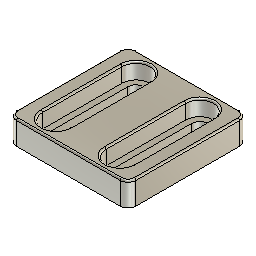
Y_stop v1_optional (Autodesk Fusion 360 design; units mm, degrees)
Autodesk Fusion 360 part; units mm, degrees
sketch "Sketch1" plane through (0, 0, 0) normal (0, 0, 1) x (1, 0, 0)
  line L0 (0, 0) -> (30, 0)
  line L1 (30, 0) -> (30, 30)
  line L2 (30, 30) -> (0, 30)
  line L3 (0, 30) -> (0, 0)
  line L4 (7, 30) -> (7, 0) construction
  line L5 (23, 30) -> (23, 0) construction
  line L6 (15, 30) -> (15, 0) construction
  line L7 (3.5, 24.986) -> (3.5, 4.986)
  line L8 (10.5, 24.986) -> (10.5, 4.986)
  arc A0 (10.5, 24.986) -> (3.5, 24.986) centre (7, 24.986) ccw
  arc A1 (3.5, 4.986) -> (10.5, 4.986) centre (7, 4.986) ccw
  line L9 (5, 24.9854) -> (5, 4.9865)
  line L10 (9, 24.986) -> (9, 4.986)
  arc A2 (9, 24.986) -> (5, 24.9854) centre (7, 24.986) ccw
  arc A3 (5, 4.9865) -> (9, 4.986) centre (7, 4.986) ccw
  line L11 (26.5, 24.986) -> (26.5, 4.986)
  line L12 (25, 24.9854) -> (25, 4.9865)
  arc A4 (25, 24.9854) -> (21, 24.986) centre (23, 24.986) ccw
  arc A5 (21, 4.986) -> (25, 4.9865) centre (23, 4.986) ccw
  arc A6 (26.5, 24.986) -> (19.5, 24.986) centre (23, 24.986) ccw
  line L13 (19.5, 24.986) -> (19.5, 4.986)
  line L14 (21, 24.986) -> (21, 4.986)
  arc A7 (19.5, 4.986) -> (26.5, 4.986) centre (23, 4.986) ccw
  point P0 (7, 21.986)
  point P1 (23, 21.9825)
  point P2 (23.0012, 7.9825)
  point P3 (7.0013, 7.986)
  point P4 (23, 21.986)
  point P5 (22.9987, 7.986)
  dimension "d1" = 30
  dimension "d2" = 30
  dimension "d3" = 16
  dimension "d4" = 14
  dimension "d5" = 7
  dimension "d6" = 3
  dimension "d7" = 14
  dimension "d8" = 16
  dimension "d9" = 7
  dimension "d10" = 3
  dimension "d11" = 7
  dimension "d12" = 4
  dimension "d13" = 4
  dimension "d14" = 4
  constraint horizontal L0
  constraint vertical L1
  constraint horizontal L2
  constraint vertical L3
  constraint coincident L0.start L3.end
  constraint parallel L1 L4
  constraint perpendicular L2 L5
  constraint coincident L2 L4.start
  constraint coincident L2 L5.start
  constraint coincident L0 L5.end
  constraint coincident L0 L4.end
  constraint coincident L4 A0.centre
  constraint coincident L4 A1.centre
  constraint midpoint L2 L6.start
  constraint midpoint L0 L6.end
  constraint perpendicular L2 L7
  constraint parallel L4 L8
  constraint symmetric L4 L7 L8
  constraint concentric A0 A2
  constraint concentric A1 A3
  constraint parallel L7 L9
  constraint parallel L4 L10
  constraint symmetric P0 L6 P4
  constraint symmetric P3 L6 P5
  constraint symmetric L6 L7.start L11.start
  constraint symmetric L6 L8.start A6.end
  constraint symmetric L6 L8.end L13.end
  constraint symmetric L6 L7.end L11.end
  constraint symmetric L6 A0 A6
  constraint symmetric L6 A1 A7
  constraint symmetric L6 L9.start L12.start
  constraint symmetric L6 L10.start A4.end
  constraint symmetric L6 L10.end A5.start
  constraint symmetric L6 L9.end L12.end
  constraint symmetric L6 A2 A4
  constraint symmetric L6 A3 A5
  measures "d1" distance of L0.start L0.end
  measures "d2" distance of L0.start L2.end
  measures "d3" distance of P2 P3
  measures "d4" distance of P1 P2
  measures "d5" diameter of A0
  measures "d6" distance of P0 A0.centre
  measures "d7" distance of P0 P3
  measures "d8" horizontal distance of P0 P1
  measures "d9" diameter of A1
  measures "d10" vertical distance of P3 A1.centre
  measures "d11" distance of L7 L8
  measures "d12" diameter of A2
  measures "d13" diameter of A3
  measures "d14" distance of L9 L10
extrude "Extrude1" add sketch "Sketch1" along normal blind 6 contours L0 L1 L2 L3
extrude "Extrude2" add sketch "Sketch1" along normal blind 2 contours L7 L8 A0 A1 | L11 A6 L13 A7
fillet "Fillet1" radius 2 4 edges at (0, 0, 3) (30, 0, 3) (30, 30, 3) (0, 30, 3)
fillet "Fillet1" radius 0.4 1 faces at (13.5, 11.6527, 6)
